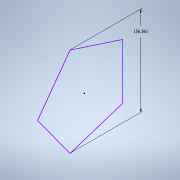
# Autodesk Inventor part: Bauteil1
Saved by Autodesk Inventor 2020.3 (Build 243373000, 373)
## iProperties
Created: 2020-05-10
Part Number: Bauteil1
Material: Generisch
Document SubType Name: Modeling
Designer: Stefan
Density: 1 g/cm^3
Appearance: Vorgabe
Author: Stefan
Autodesk Inventor part; units mm, degrees
ref_plane "YZ Plane" through (0, 0, 0) normal (1, 0, 0) x (0, 1, 0)
ref_plane "XZ Plane" through (0, 0, 0) normal (0, 1, 0) x (-1, 0, 0)
ref_plane "XY Plane" through (0, 0, 0) normal (0, 0, 1) x (1, 0, 0)
sketch "Skizze1" plane through (0, 0, 0) normal (1, 0, 0) x (0, 1, 0)
  line L0 (0, 83.1323) -> (79.0635, 25.6893)
  line L1 (79.0635, 25.6893) -> (48.8639, -67.2554)
  line L2 (48.8639, -67.2554) -> (-48.8639, -67.2554)
  line L3 (-48.8639, -67.2554) -> (-79.0635, 25.6893)
  line L4 (-79.0635, 25.6893) -> (0, 83.1323)
  line L5 (0, 62.103) -> (59.0635, 19.1909)
  line L6 (59.0635, 19.1909) -> (36.5033, -50.2424)
  line L7 (36.5033, -50.2424) -> (-36.5033, -50.2424)
  line L8 (-36.5033, -50.2424) -> (-59.0635, 19.1909)
  line L9 (-59.0635, 19.1909) -> (0, 62.103)
  point P0 (0, 0)
  point P1 (0, 0)
  point P2 (0, 0)
  dimension "d0" = 158.127
  dimension "d4" = 118.127
  constraints: 20 end point, 2 coincident, 22 other
  measures "d0" distance of L0.end L3.end
  measures "d4" distance of L5.end L8.end
extrude "Extrusion2" add sketch "Skizze1" along normal blind 4
